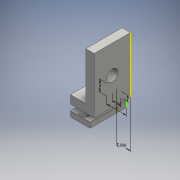
# Autodesk Inventor part: bloceur_alim
Saved by Autodesk Inventor 2016 (Build 200138000, 138)
## iProperties
Created: 2018-12-10
Part Number: bloceur_alim
Material: Generic
Document SubType Name: Modeling
Designer: Mick
Density: 1 g/cm^3
Appearance: Default
Author: Mick
Autodesk Inventor part; units mm, degrees
ref_plane "YZ Plane" through (0, 0, 0) normal (1, 0, 0) x (0, 1, 0)
ref_plane "XZ Plane" through (0, 0, 0) normal (0, 1, 0) x (-1, 0, 0)
ref_plane "XY Plane" through (0, 0, 0) normal (0, 0, 1) x (1, 0, 0)
sketch "Sketch1" plane through (0, 0, 0) normal (0, 1, 0) x (-1, 0, 0)
  line L0 (0, 0) -> (3, 0)
  line L1 (3, 0) -> (3, -20)
  line L2 (3, -20) -> (0, -20)
  line L3 (0, -20) -> (0, 0)
  line L4 (3, -20) -> (16, -20)
  line L5 (16, -20) -> (16, -17)
  line L6 (16, -17) -> (3, -17)
  line L7 (3, -17) -> (3, -20)
  dimension "d0" = 3
  dimension "d1" = 20
  dimension "d2" = 13
  dimension "d3" = 3
  constraints: 16 end point, 4 parallel, 2 horizontal, 2 perpendicular
  measures "d0" distance of L1.end L2.end
  measures "d1" distance of L0.end L1.end
  measures "d2" distance of L6.end L5.end
  measures "d3" distance of L5.end L4.end
extrude "Extrusion1" add sketch "Sketch1" against normal blind 13
sketch "Sketch2" plane through (0, 0, 0) normal (0, 1, 0) x (1, 0, 0)
  line L0 (-16, 20) -> (0, 20) projected
  line L1 (0, 0) -> (0, 20) projected
  line L2 (-6.3982, 20) -> (-3.3982, 20)
  line L3 (-3.3982, 20) -> (-3.3982, 22)
  line L4 (-3.3982, 22) -> (-6.3982, 22)
  line L5 (-6.3982, 22) -> (-6.3982, 20)
  line L6 (-6.3982, 20) -> (-3.3982, 22) construction
  line L7 (-6.3982, 22) -> (-3.3982, 20) construction
  line L8 (0, 20) -> (-16, 20) projected
  line L9 (-1.4593, 20) -> (-8.4593, 20)
  line L10 (-8.4593, 20) -> (-8.4593, 24)
  line L11 (-8.4593, 24) -> (-1.4593, 24)
  line L12 (-1.4593, 24) -> (-1.4593, 20)
  line L13 (-8.4593, 22) -> (-1.4593, 22)
  point P0 (-4.8982, 20)
  point P1 (-4.8982, 21)
  dimension "d6" = 4.8982
  dimension "d7" = 3
  dimension "d8" = 2
  dimension "d9" = 7
  dimension "d10" = 4
  constraints: 22 end point, 4 parallel, 3 midpoint, 2 horizontal, 2 perpendicular, 2 point on line, 1 collinear
  measures "d6" distance from line of point (-4.898, 20) L1
  measures "d7" distance of L4.end L3.end
  measures "d8" distance of L3.end L2.end
  measures "d9" distance of L10.end L11.end
  measures "d10" distance of L9.end L10.end
extrude "Extrusion2" add sketch "Sketch2" against normal up to surface (13 mm away) contours L5 L4 L3 L0
extrude "Extrusion3" add sketch "Sketch2" against normal blind 2
extrude "Extrusion4" add sketch "Sketch2" against normal up to surface (13 mm away) contours L10 L11 L12 L13 L4
fillet "Fillet1" radius 1.5 2 edges at (-6.3982, -13, -21) (-3.3982, -13, -21)
sketch "Sketch3" plane through (0, 0, 0) normal (0, 1, 0) x (1, 0, 0)
  line L0 (-16, 17) -> (-3, 17) projected
  line L1 (-8.4593, 20) -> (-16, 20) projected
  line L2 (-16, 17) -> (-8.4593, 17)
  line L3 (-8.4593, 17) -> (-8.4593, 20)
  line L4 (-8.4593, 20) -> (-16, 20)
  line L5 (-16, 20) -> (-16, 17)
  point P0 (0, 0)
  constraints: 8 end point, 2 parallel, 1 horizontal, 1 perpendicular
extrude "Extrusion5" cut sketch "Sketch3" against normal up to next
sketch "Sketch7" plane through (-3, 0, -17) normal (-1, 0, 0) x (0, 0, 1)
  line L0 (0, 0) -> (17, 0) projected
  line L1 (17, 0) -> (17, -13) projected
  point P0 (7, -6.5)
  dimension "d41" = 6.5
  dimension "d42" = 10
  measures "d41" distance from line of point (7, -6.5) L0
  measures "d42" distance from line of point (7, -6.5) L1
hole "Hole2" at (-3, -6.5, -10) direction (1, 0, 0) diameter 4 end through all
body "Solid1"
